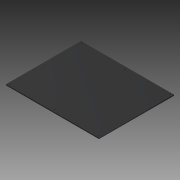
# Autodesk Inventor part: ElectronicsLowerPanel
Saved by Autodesk Inventor 2015 SP1 (Build 190203100, 203)
## iProperties
Category: Panel
Created: 2015-01-14
Part Number: ElectronicsLowerPanel
Material: ABS Plastic
Document SubType Name: Modeling
Designer: Jack
Density: 1.06 g/cm^3
Appearance: Smooth - Dark Gray
Mass: 818.214 g
Surface Area: 3929.9 cm^2
Volume: 771.9 cm^3
Vendor: Tap Plastics
Author: Jack
Autodesk Inventor part; units mm, degrees
ref_plane "YZ Plane" through (0, 0, 0) normal (1, 0, 0) x (0, 1, 0)
ref_plane "XZ Plane" through (0, 0, 0) normal (0, 1, 0) x (-1, 0, 0)
ref_plane "XY Plane" through (0, 0, 0) normal (0, 0, 1) x (1, 0, 0)
sketch "Sketch1" plane through (0, 0, 0) normal (0, 0, 1) x (1, 0, 0)
  line L0 (0, 0) -> (465, 0)
  line L1 (465, 0) -> (465, 375)
  line L2 (465, 375) -> (0, 375)
  line L3 (0, 375) -> (0, 0)
  dimension "d0" = 465
  dimension "d1" = 375
  constraints: 8 end point, 2 parallel, 1 horizontal, 1 perpendicular
  measures "d0" distance of L2.end L1.end
  measures "d1" distance of L1.end L0.end
extrude "Extrusion1" add sketch "Sketch1" along normal blind 4.7625
sketch "Sketch2" plane through (0, 0, 4.7625) normal (0, 0, 1) x (1, 0, 0)
  line L0 (0, 0) -> (465, 0) projected
  line L1 (465, 0) -> (465, 375) projected
  line L2 (465, 375) -> (0, 375) projected
  line L3 (0, 375) -> (0, 0) projected
  point P0 (12, 367.5)
  point P1 (232.5, 363)
  point P2 (12, 7.5)
  point P3 (232.5, 12)
  point P4 (453, 7.5)
  point P5 (453, 367.5)
  dimension "d4" = 7.5
  dimension "d5" = 12
  dimension "d6" = 7.5
  dimension "d7" = 12
  dimension "d8" = 232.5
  dimension "d16" = 12
  dimension "d17" = 12
  constraints: 3 vertical alignment, 2 horizontal alignment
  measures "d4" distance from line of L0 point (12, 7.5)
  measures "d5" distance from line of L3 point (12, 7.5)
  measures "d6" distance from line of L2 point (12, 367.5)
  measures "d7" distance from line of L1 point (453, 367.5)
  measures "d8" distance from line of L1 point (232.5, 12)
  measures "d16" distance from line of L0 point (232.5, 12)
  measures "d17" distance from line of L2 point (232.5, 363)
hole "Hole1" at (12, 367.5, 4.7625) at (232.5, 363, 4.7625) at (12, 7.5, 4.7625) at (232.5, 12, 4.7625) at (453, 7.5, 4.7625) at (453, 367.5, 4.7625) direction (0, 0, -1) diameter 5 end through all
body "Solid1"
